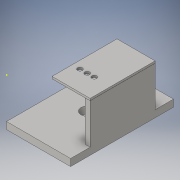
# Autodesk Inventor part: Part3
Saved by Autodesk Inventor 2016 (Build 200138000, 138)
## iProperties
Created: 2016-03-23
Part Number: Part3
Material: Generic
Document SubType Name: Modeling
Designer: Dhivya Sukumar
Density: 1 g/cm^3
Appearance: Default
Author: Dhivya Sukumar
Autodesk Inventor part; units mm, degrees
note: some values were not read from the file. Chosen so that the rebuilt part matches the saved one: direction of "Hole1".
ref_plane "YZ Plane" through (0, 0, 0) normal (1, 0, 0) x (0, 1, 0)
ref_plane "XZ Plane" through (0, 0, 0) normal (0, 1, 0) x (-1, 0, 0)
ref_plane "XY Plane" through (0, 0, 0) normal (0, 0, 1) x (1, 0, 0)
sketch "Sketch1" plane through (0, 0, 0) normal (0, 1, 0) x (-1, 0, 0)
  line L0 (0, 0) -> (-63.7459, 0)
  line L1 (-63.7459, 0) -> (-63.7459, -102.4121)
  line L2 (-63.7459, -102.4121) -> (0, -102.4121)
  line L3 (0, -102.4121) -> (0, 0)
  line L4 (-57.4973, -89.9149) -> (-63.7459, -89.9149)
  line L5 (-63.7459, -89.9149) -> (-63.7459, -20.7341)
  circle A0 centre (-31.873, -51.2061) radius 6.35
  constraints: 12 end point, 2 parallel, 1 centre point, 1 horizontal, 1 perpendicular, 1 point on line
extrude "Extrusion1" add sketch "Sketch1" along normal blind 7 contours L3 L2 L1 L0 | A0
sketch "Sketch2" plane through (0, 7, 0) normal (0, 1, 0) x (1, 0, 0)
  line L0 (63.7459, 0) -> (63.7459, 102.4121) projected
  line L1 (63.7459, 19.5256) -> (58.7459, 19.5256)
  line L2 (58.7459, 19.5256) -> (58.7459, 84.196)
  line L3 (58.7459, 84.196) -> (63.7459, 84.196)
  line L4 (63.7459, 84.196) -> (63.7459, 19.5256)
  point P0 (0, 0)
  dimension "d37" = 5
  constraints: 8 end point, 2 parallel, 1 horizontal, 1 perpendicular, 1 point on line
  measures "d37" distance of L2.end L3.end
extrude "Extrusion2" add sketch "Sketch2" along normal blind 40
sketch "Sketch3" plane through (0, 47, 0) normal (0, 1, 0) x (1, 0, 0)
  point P0 (0, 0)
sketch "Sketch4" plane through (0, 47, 0) normal (0, 1, 0) x (1, 0, 0)
  line L0 (63.6489, 19.5244) -> (25.7429, 19.5244)
  line L1 (25.7429, 19.5244) -> (25.7429, 84.2091)
  line L2 (25.7429, 84.2091) -> (63.6489, 84.2091)
  line L3 (63.6489, 84.2091) -> (63.6489, 19.5244)
  point P0 (0, 0)
  constraints: 8 end point, 2 parallel, 1 horizontal, 1 perpendicular
extrude "Extrusion3" add sketch "Sketch4" along normal blind 2
hole "Hole1" at (33.3915, 49, -39.6826) direction (0, -1, 0) diameter 4.826 end up to surface
hole "Hole2" at (40.6045, 49, -39.7222) direction (0, -1, 0) diameter 4.826 depth 4.7625
hole "Hole3" at (47.4379, 49, -39.912) direction (0, -1, 0) diameter 4.826 depth 4.7625
hole "Hole4" at (31.3368, 0, -49.1509) direction (0, 1, 0) diameter 12.7 depth 7.725
body "Solid1"
